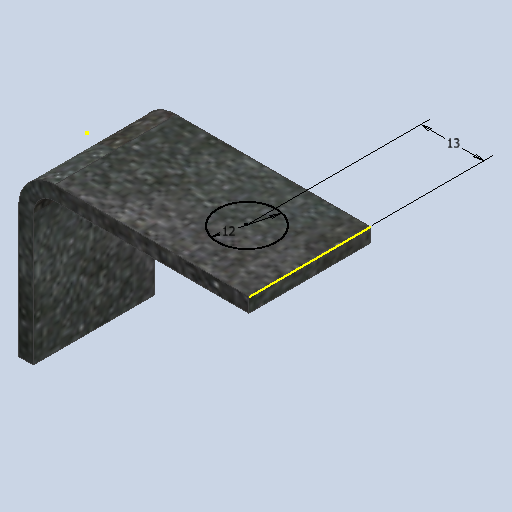
# Autodesk Inventor part: clampBaseTopSide
Saved by Autodesk Inventor 2024.2 (Build 282272000, 272)
## iProperties
Created: 2024-05-25
Part Number: clampBaseTopSide
Material: Steel
Document SubType Name: Modeling
Designer: user
Density: 7.85 g/cm^3
Appearance: Plate
Author: user
Autodesk Inventor part; units mm, degrees
ref_plane "XZ Plane" through (0, 0, 0) normal (0, 1, 0) x (-1, 0, 0)
ref_plane "XY Plane" through (0, 0, 0) normal (0, 0, 1) x (1, 0, 0)
sketch "Sketch1" plane through (0, 0, 0) normal (0, 0, 1) x (1, 0, 0)
  line L0 (0, 0) -> (0, 27)
  line L1 (6, 33) -> (46, 33)
  arc A0 (6, 33) -> (0, 27) centre (6, 27) ccw
  point P0 (0, 33)
  dimension "d0" = 33
  dimension "d1" = 46
  dimension "d4" = 6
  constraints: 4 end point, 2 point on circle, 2 point on line, 2 tangent, 1 centre point, 1 perpendicular, 1 vertical
  measures "d0" distance of L0.start point (0, 33)
  measures "d1" distance of point (0, 33) L1.end
  measures "d4" radius of A0
sketch "Sketch2" plane through (0, 0, 0) normal (0, 1, 0) x (-1, 0, 0)
  line L0 (-1.5, -12.5) -> (1.5, -12.5)
  line L1 (1.5, -12.5) -> (1.5, 12.5)
  line L2 (1.5, 12.5) -> (-1.5, 12.5)
  line L3 (-1.5, 12.5) -> (-1.5, -12.5)
  line L4 (-1.5, -12.5) -> (1.5, 12.5) construction
  line L5 (1.5, -12.5) -> (-1.5, 12.5) construction
  point P0 (0, 0)
  dimension "d2" = 3
  dimension "d3" = 25
  constraints: 12 end point, 2 midpoint, 2 parallel, 1 horizontal, 1 perpendicular
  measures "d2" distance of L2.end L1.end
  measures "d3" distance of L1.end L0.end
sweep "Sweep1" add profiles "Sketch2" path "Sketch1"
sketch "Sketch3" plane through (6, 34.5, 12.5) normal (0, 1, 0) x (1, 0, 0)
  circle A0 centre (27, 12.5) radius 6
  line L0 (40, 25) -> (40, 0) projected
  point P0 (-6, 12.5)
  dimension "d7" = 12
  dimension "d8" = 13
  constraints: 1 centre point, 1 horizontal alignment
  measures "d7" diameter of A0
  measures "d8" distance from line of L0 A0.centre
ref_plane "Work Plane1" through (33, 0, 0) normal (1, 0, 0) x (0, 1, 0)
body "Solid1"
